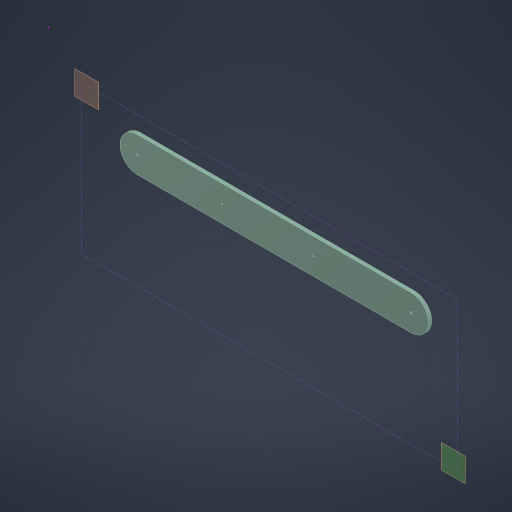
# Autodesk Inventor part: foot1
Saved by Autodesk Inventor 2024.2 (Build 282272000, 272)
## iProperties
Created: 2024-06-20
Part Number: foot1
Material: Generic
Document SubType Name: Modeling
Designer: Moe
Density: 1 g/cm^3
Appearance: Default
Author: Moe
Autodesk Inventor part; units mm, degrees
ref_plane "YZ Plane" through (0, 0, 0) normal (1, 0, 0) x (0, 1, 0)
ref_plane "XZ Plane" through (0, 0, 0) normal (0, 1, 0) x (-1, 0, 0)
ref_plane "XY Plane" through (0, 0, 0) normal (0, 0, 1) x (1, 0, 0)
ref_plane "Work Plane2" through (35.545, -31.609, 1.6) normal (0, 0, 1) x (1, 0, 0)
sketch "Sketch2" plane through (35.545, -31.609, 1.6) normal (0, 0, 1) x (1, 0, 0)
  line L0 (-4.7778, 3.1171) -> (341.5466, 3.1925) construction
  line L1 (341.5466, 3.1925) -> (341.5765, -133.848) construction
  line L2 (341.5765, -133.848) -> (-4.7479, -133.9235) construction
  line L3 (-4.7479, -133.9235) -> (-4.7778, 3.1171) construction
  point P0 (-35.545, 31.609)
  constraints: 2 other
ref_plane "Work Plane1" through (371.545, -162.609, 0) normal (0, 0, -1) x (-1, 0, 0)
ref_plane "Work Plane3" through (371.545, -162.609, 0) normal (0, 0, 1) x (1, 0, 0)
sketch "Sketch10" plane through (371.545, -162.609, 0) normal (0, 0, 1) x (1, 0, 0)
  line L0 (-288.039, 119.527) -> (-35.979, 119.527)
  line L1 (-19.979, 103.527) -> (-19.979, 103.527)
  line L2 (-35.979, 87.527) -> (-288.039, 87.527)
  line L3 (-304.039, 103.527) -> (-304.039, 103.527)
  circle A0 centre (-288.039, 103.527) radius 1.1 projected
  circle A1 centre (-35.979, 103.44) radius 1.1 projected
  arc A2 (-19.979, 103.527) -> (-35.979, 119.527) centre (-35.979, 103.527) ccw
  arc A3 (-35.979, 87.527) -> (-19.979, 103.527) centre (-35.979, 103.527) ccw
  arc A4 (-304.039, 103.527) -> (-288.039, 87.527) centre (-288.039, 103.527) ccw
  arc A5 (-288.039, 119.527) -> (-304.039, 103.527) centre (-288.039, 103.527) ccw
  circle A6 centre (-210.039, 103.527) radius 1.1 projected
  circle A7 centre (-125.979, 103.44) radius 1.1 projected
  point P0 (-371.545, 162.609)
  dimension "d89" = 16
  dimension "d91" = 16
  dimension "d92" = 16
  dimension "d93" = 16
  dimension "d94" = 16
  constraints: 8 end point, 8 point on circle, 8 tangent, 4 centre point, 3 equal radius, 2 parallel, 1 horizontal, 1 perpendicular
  measures "d89" distance from line of L0 A0.centre
  measures "d91" distance from line of L2 A0.centre
  measures "d92" distance from line of A0.centre L3
  measures "d93" distance from line of L1 A1.centre
  measures "d94" radius of A2
extrude "Extrusion5" add sketch "Sketch10" along normal blind 3
body "Solid1"
